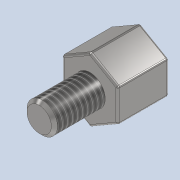
# Autodesk Inventor part: hexagonal_spacer_M3_5mm
Saved by Autodesk Inventor 2022 (Build 260153000, 153)
## iProperties
Created: 2021-08-05
Part Number: hexagonal_spacer_M3_5mm
Material: 鋼、炭素鋼
Document SubType Name: Modeling
Designer: yuta0
Density: 7.85 g/cm^3
Appearance: 半つや出し
購入先: 西川電子
在庫数: 0.0
Author: yuta0
Autodesk Inventor part; units mm, degrees
ref_plane "YZ Plane" through (0, 0, 0) normal (1, 0, 0) x (0, 1, 0)
ref_plane "XZ Plane" through (0, 0, 0) normal (0, 1, 0) x (-1, 0, 0)
ref_plane "XY Plane" through (0, 0, 0) normal (0, 0, 1) x (1, 0, 0)
sketch "スケッチ1" plane through (0, 0, 0) normal (0, 0, 1) x (1, 0, 0)
  line L0 (0, 3.1754) -> (2.75, 1.5877)
  line L1 (2.75, 1.5877) -> (2.75, -1.5877)
  line L2 (2.75, -1.5877) -> (0, -3.1754)
  line L3 (0, -3.1754) -> (-2.75, -1.5877)
  line L4 (-2.75, -1.5877) -> (-2.75, 1.5877)
  line L5 (-2.75, 1.5877) -> (0, 3.1754)
  point P0 (0, 0)
  point P1 (0, 0)
  dimension "d0" = 5.5
  constraints: 12 end point, 1 coincident, 13 other
  measures "d0" distance between parallel lines of L4 L1
extrude "押し出し1" add sketch "スケッチ1" along normal blind 5
sketch "スケッチ2" plane through (0, 0, 5) normal (0, 0, 1) x (1, 0, 0)
  circle A0 centre (0, 0) radius 1.5
  dimension "d3" = 3
  constraints: 1 centre point, 1 coincident
  measures "d3" diameter of A0
extrude "押し出し2" add sketch "スケッチ2" along normal blind 5
thread "ねじ1" size "M3x0.5" class "6g" standard "ANSI Metric M Profile" length 12
chamfer "面取り1" distance 0.3 angle 45 1 edges at (-1.5, 0, 10)
fillet "フィレット1" radius 0.2 18 edges at (-1.375, 2.3816, 5) (1.375, 2.3816, 5) (2.75, 0, 5) (1.375, -2.3816, 5) (-1.375, -2.3816, 5) (-2.75, 0, 5) (-2.75, -1.5877, 2.5) (0, -3.1754, 2.5) (2.75, -1.5877, 2.5) (2.75, 1.5877, 2.5) (0, 3.1754, 2.5) (-2.75, 1.5877, 2.5) (-1.375, 2.3816, 0) (1.375, 2.3816, 0) (2.75, 0, 0) (1.375, -2.3816, 0) (-1.375, -2.3816, 0) (-2.75, 0, 0)
sketch "スケッチ3" plane through (0, 0, 0) normal (0, 0, -1) x (-1, 0, 0)
  point P0 (0, 0)
hole "穴1" at (0, 0, 0) direction (0, 0, 1) diameter 2.459 depth 5 tip angle 118 thread size "M3x0.5" class "6H" standard "ANSI Metric M Profile"
chamfer "面取り2" distance 0.2 angle 45 1 edges at (0, -1.2295, 0)
